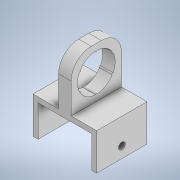
# Autodesk Inventor part: Eje_Carril
Saved by Autodesk Inventor 2022 (Build 260153000, 153)
## iProperties
Created: 2022-02-07
Part Number: Eje_Carril
Material: Generic
Document SubType Name: Modeling
Designer: katha
Density: 1 g/cm^3
Appearance: Default
Author: katha
Autodesk Inventor part; units mm, degrees
ref_plane "YZ Plane" through (0, 0, 0) normal (1, 0, 0) x (0, 1, 0)
ref_plane "XZ Plane" through (0, 0, 0) normal (0, 1, 0) x (-1, 0, 0)
ref_plane "XY Plane" through (0, 0, 0) normal (0, 0, 1) x (1, 0, 0)
sketch "Sketch2" plane through (0, 0, 0) normal (0, 0, 1) x (1, 0, 0)
  line L0 (31.3357, -4.795) -> (6.3357, -4.795) projected
  line L1 (6.3357, -4.795) -> (6.3357, -1.5952) projected
  line L2 (31.3357, -1.5952) -> (6.3357, -1.5952) projected
  line L3 (31.3357, -4.795) -> (31.3357, -1.5952) projected
  line L4 (6.3357, -1.5952) -> (6.3357, -21.5944) projected
  line L5 (6.3357, -21.5944) -> (3.1357, -21.5944) projected
  line L6 (3.1357, -1.5952) -> (3.1357, -21.5944) projected
  line L7 (6.3357, -1.5952) -> (3.1357, -1.5952) projected
  line L8 (31.3357, -21.5944) -> (31.3357, -1.5952) projected
  line L9 (31.3357, -1.5952) -> (34.5357, -1.5952) projected
  line L10 (34.5357, -21.5944) -> (34.5357, -1.5952) projected
  line L11 (31.3357, -21.5944) -> (34.5357, -21.5944) projected
  line L12 (6.3357, -23.8087) -> (3.1357, -23.8087) projected
  line L13 (34.8357, -21.5944) -> (34.8357, -2.6826)
  line L14 (34.8357, -21.5944) -> (37.8357, -21.5944)
  line L15 (37.8357, -21.5944) -> (37.8357, 0.3174)
  line L16 (18.8357, -1.5952) -> (18.8357, -12.9026) construction
  line L17 (2.8357, -21.5944) -> (2.8357, -2.6826)
  line L18 (2.8357, -21.5944) -> (-0.1643, -21.5944)
  line L19 (-0.1643, -21.5944) -> (-0.1643, 0.3174)
  line L20 (2.8357, -2.6826) -> (34.8357, -2.6826)
  line L21 (-0.1643, 0.3174) -> (37.8357, 0.3174)
  line L22 (22.5857, 0.3174) -> (22.5857, 30.3174)
  line L23 (22.5857, 30.3174) -> (15.0857, 30.3174)
  line L24 (15.0857, 30.3174) -> (15.0857, 0.3174)
  line L25 (6.3357, -2.9826) -> (31.3357, -2.9826) projected
  point P0 (0, 0)
  dimension "d1" = 0.3
  dimension "d2" = 3
  dimension "d5" = 32
  dimension "d9" = 30
  dimension "d10" = 7.5
  dimension "d11" = 3.75
  dimension "d18" = 0.3
  dimension "d19" = 3
  constraints: 24 end point, 3 horizontal, 3 perpendicular, 3 symmetric about line, 2 point on line, 2 vertical, 1 collinear, 1 midpoint
  measures "d1" distance between parallel lines of L10 L13
  measures "d2" distance of L13.start L14.end
  measures "d5" distance of L13.end L17.end
  measures "d9" distance of L22.start L22.end
  measures "d10" distance of L22.end L23.end
  measures "d11" distance between parallel lines of L16 L22
  measures "d18" vertical distance of L13.end L25.end
  measures "d19" distance between parallel lines of L21 L20
extrude "Extrusion1" add sketch "Sketch2" along normal mid plane 30 contours L20 L1 L2 L3 | L3 L9 L10 L20 | L20 L6 L7 L1 | L2 L7 L6 L20 L17 L18 L19 L21 L15 L14 L13 L10 L9 | L21 L24 L23 L22
sketch "Sketch3" plane through (37.8357, -21.5944, 15) normal (1, 0, 0) x (0, 0, -1)
  circle A0 centre (13.5169, 6.5933) radius 2 projected
  line L0 (30, 21.9118) -> (30, 0) projected
  line L1 (0, 0) -> (0, 21.9118) projected
  line L2 (30, 0) -> (0, 0) projected
  line L3 (0, 21.9118) -> (30, 21.9118) projected
  line L4 (30, 0) -> (0, 0) projected
  line L5 (15, 0) -> (15, 21.9118) construction
  circle A1 centre (15, 6.5933) radius 2
  point P0 (15, 21.5944)
  dimension "d14" = 4
  dimension "d15" = 6.5933
  constraints: 2 end point, 2 midpoint, 1 centre point, 1 point on line
  measures "d14" diameter of A1
  measures "d15" distance from line of L2 A1.centre
extrude "Extrusion2" cut sketch "Sketch3" against normal blind 60 contours A0 A1 | A0 A1 picked at (14.6591, 6.7506) picked at (16.4859, 6.7542)
sketch "Sketch4" plane through (15.0857, 0.3174, 15) normal (-1, 0, 0) x (0, 0, 1)
  line L0 (-30, 0) -> (0, 0) projected
  line L1 (0, 30) -> (0, 0) projected
  line L2 (-30, 30) -> (0, 30) projected
  line L3 (-30, 0) -> (-30, 30) projected
  line L4 (-30, 0) -> (0, 0) projected
  line L5 (-15, 0) -> (-15, 30) construction
  line L6 (-30, 30) -> (0, 30) projected
  line L7 (0, 0) -> (0, 30) projected
  line L8 (0, 15) -> (-30, 15) construction
  circle A0 centre (-15, 15) radius 11.25
  arc A1 (-14.5001, 3.7611) -> (-15.4999, 3.7611) centre (-15, 3.75) ccw
  arc A2 (-5.0169, 9.8135) -> (-5.5168, 8.9476) centre (-5.2572, 9.375) ccw
  arc A3 (-5.5168, 21.0524) -> (-5.0169, 20.1865) centre (-5.2572, 20.625) ccw
  arc A4 (-15.4999, 26.2389) -> (-14.5001, 26.2389) centre (-15, 26.25) ccw
  arc A5 (-24.9831, 20.1865) -> (-24.4832, 21.0524) centre (-24.7428, 20.625) ccw
  arc A6 (-24.4832, 8.9476) -> (-24.9831, 9.8135) centre (-24.7428, 9.375) ccw
  point P0 (-15, -0.3174)
  point P1 (-24.9831, 9.8135)
  point P2 (-24.4832, 8.9476)
  point P3 (-5.5168, 8.9476)
  point P4 (-5.0169, 9.8135)
  point P5 (-5.0169, 20.1865)
  point P6 (-5.5168, 21.0524)
  point P7 (-14.5001, 26.2389)
  point P8 (-15.4999, 26.2389)
  point P9 (-24.4832, 21.0524)
  point P10 (-24.9831, 20.1865)
  dimension "d20" = 22.5
  dimension "d21" = 1
  dimension "d24" = 360
  constraints: 15 point on circle, 7 centre point, 5 midpoint, 4 end point, 1 point on line, 25 other
  measures "d20" diameter of A0
  measures "d21" diameter of A1
extrude "Extrusion3" cut sketch "Sketch4" against normal blind 10 contours A0 A2 A1 A6 A5 A4 A3
fillet "Fillet1" radius 12 2 edges at (18.8357, 30.3174, 15) (18.8357, 30.3174, -15)
body "Solid1"
